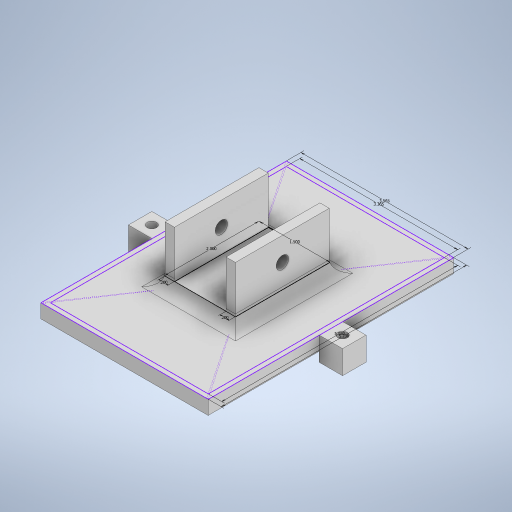
# Autodesk Inventor part: HotplateRetainer for 8020
Saved by Autodesk Inventor 2024.1 (Build 281209000, 209)
## iProperties
Created: 2022-02-14
Part Number: HotplateRetainer for 8020
Material: Generic
Document SubType Name: Modeling
Designer: Beaucage
Density: 1 g/cm^3
Appearance: Default
Author: Beaucage
Autodesk Inventor part; units mm, degrees
ref_plane "YZ Plane" through (0, 0, 0) normal (1, 0, 0) x (0, 1, 0)
ref_plane "XZ Plane" through (0, 0, 0) normal (0, 1, 0) x (-1, 0, 0)
ref_plane "XY Plane" through (0, 0, 0) normal (0, 0, 1) x (1, 0, 0)
sketch "Sketch1" plane through (0, 0, 0) normal (0, 1, 0) x (-1, 0, 0)
  line L0 (0, 0) -> (38.1, 0)
  line L1 (38.1, 0) -> (38.1, -50.8)
  line L2 (38.1, -50.8) -> (0, -50.8)
  line L3 (0, -50.8) -> (0, 0)
  line L4 (38.1, -50.8) -> (33.02, -50.8)
  line L5 (33.02, -50.8) -> (33.02, 0)
  line L6 (33.02, 0) -> (38.1, 0)
  line L7 (38.1, 0) -> (38.1, -50.8)
  line L8 (0, -50.8) -> (5.08, -50.8)
  line L9 (5.08, -50.8) -> (5.08, 0)
  line L10 (5.08, 0) -> (0, 0)
  line L11 (0, 0) -> (0, -50.8)
  dimension "d0" = 38.1
  dimension "d1" = 50.8
  dimension "d2" = 5.08
  dimension "d3" = 5.08
  constraints: 24 end point, 6 parallel, 3 horizontal, 3 perpendicular, 2 point on line
  measures "d0" distance of L1.end L2.end
  measures "d1" distance of L0.end L1.end
  measures "d2" distance of L5.end L6.end
  measures "d3" distance of L10.end L9.end
extrude "Extrusion1" add sketch "Sketch1" along normal blind 25.4 contours L0 L9 L2 L3 | L0 L1 L2 L5
extrude "Extrusion2" add sketch "Sketch1" against normal blind 5.08
sketch "Sketch2" plane through (0, 25.4, 0) normal (1, 0, 0) x (0, 0, -1)
  line L0 (50.8, 0) -> (0, 0) projected
  line L1 (25.4, 0) -> (25.4, -12.7)
  point P0 (0, -25.4)
  dimension "d8" = 12.7
  constraints: 2 end point, 1 midpoint, 1 vertical
  measures "d8" distance of L1.start L1.end
hole "Hole1" at (0, 12.7, -25.4) direction (-1, 0, 0) diameter 6.7564 end through all start extended yes clearance for "Socket Head Cap Screw" size "1/4" standard "Ansi Unified Screw Threads"
sketch "Sketch3" plane through (0, -5.08, 0) normal (0, -1, 0) x (1, 0, 0)
  line L0 (0, 0) -> (-38.1, 0) projected
  line L1 (-38.1, 0) -> (-38.1, -50.8) projected
  line L2 (-38.1, -50.8) -> (0, -50.8) projected
  line L3 (0, -50.8) -> (0, 0) projected
  line L4 (-61.7906, 38.4797) -> (23.6906, 38.4797)
  line L5 (23.6906, 38.4797) -> (23.6906, -89.2797)
  line L6 (23.6906, -89.2797) -> (-61.7906, -89.2797)
  line L7 (-61.7906, -89.2797) -> (-61.7906, 38.4797)
  line L8 (-61.7906, 38.4797) -> (23.6906, -89.2797) construction
  line L9 (23.6906, 38.4797) -> (-61.7906, -89.2797) construction
  line L10 (-63.4909, 41.021) -> (25.3909, 41.021)
  line L11 (25.3909, -91.821) -> (-63.4909, -91.821)
  line L12 (-63.4909, 41.021) -> (25.3909, -91.821) construction
  line L13 (25.3909, 41.021) -> (-63.4909, -91.821) construction
  line L14 (-64.3255, 41.021) -> (26.2255, 41.021)
  line L15 (26.2255, 41.021) -> (26.2255, -91.821)
  line L16 (26.2255, -91.821) -> (-64.3255, -91.821)
  line L17 (-64.3255, -91.821) -> (-64.3255, 41.021)
  line L18 (-64.3255, 41.021) -> (26.2255, -91.821) construction
  line L19 (26.2255, 41.021) -> (-64.3255, -91.821) construction
  point P0 (-19.05, -25.4)
  point P1 (25.3909, 41.021)
  dimension "d16" = 85.4812
  dimension "d17" = 127.7595
  dimension "d18" = 132.842
  dimension "d19" = 90.551
  constraints: 32 end point, 6 midpoint, 5 parallel, 3 horizontal, 2 perpendicular
  measures "d16" distance of L5.end L6.end
  measures "d17" distance of L4.end L5.end
  measures "d18" distance of L10.end L11.start
  measures "d19" distance of L15.end L16.end
extrude "Extrusion3" add sketch "Sketch3" along normal blind 2.54 contours L3 L2 L1 L0 | L4 L5 L6 L7
extrude "Extrusion4" add sketch "Sketch3" along normal blind 7.62 contours L10 L14 L15 L16 L11 L17
fillet "Fillet1" radius 6.35 4 edges at (-38.1, -5.08, -25.4) (-19.05, -5.08, -50.8) (0, -5.08, -25.4) (-19.05, -5.08, 0)
sketch "Sketch4" plane through (0, -5.08, 0) normal (0, 1, 0) x (1, 0, 0)
  line L0 (-51.6255, 19.05) -> (-77.0255, 19.05)
  line L1 (-77.0255, 19.05) -> (-77.0255, 31.75)
  line L2 (-77.0255, 31.75) -> (-51.6255, 31.75)
  line L3 (-51.6255, 31.75) -> (-51.6255, 19.05)
  line L4 (-64.3255, -41.021) -> (-64.3255, 91.821) projected
  line L5 (-51.6255, 19.05) -> (-77.0255, 31.75) construction
  line L6 (-77.0255, 19.05) -> (-51.6255, 31.75) construction
  line L7 (13.5255, 19.05) -> (38.9255, 19.05)
  line L8 (38.9255, 19.05) -> (38.9255, 31.75)
  line L9 (38.9255, 31.75) -> (13.5255, 31.75)
  line L10 (13.5255, 31.75) -> (13.5255, 19.05)
  line L11 (26.2255, 91.821) -> (26.2255, -41.021) projected
  line L12 (13.5255, 19.05) -> (38.9255, 31.75) construction
  line L13 (38.9255, 19.05) -> (13.5255, 31.75) construction
  point P0 (0, 0)
  point P1 (-64.3255, 25.4)
  point P2 (26.2255, 25.4)
  point P3 (26.2255, 31.75)
  point P4 (26.2255, 19.05)
  point P5 (-64.3255, 19.05)
  point P6 (-64.3255, 31.75)
  dimension "d25" = 25.4
  dimension "d26" = 12.7
  dimension "d27" = 25.4
  dimension "d28" = 12.7
  constraints: 24 end point, 6 midpoint, 4 parallel, 2 horizontal, 2 perpendicular
  measures "d25" distance of L1.end L2.end
  measures "d26" distance of L0.end L1.end
  measures "d27" distance of L9.end L8.end
  measures "d28" distance of L8.end L7.end
extrude "Extrusion5" add sketch "Sketch4" against normal blind 12.7 contours L0 L1 L2 L4 | L11 L9 L8 L7
sketch "Sketch5" plane through (0, -17.78, 0) normal (0, -1, 0) x (1, 0, 0)
  line L0 (26.2255, -31.75) -> (38.9255, -31.75) projected
  line L1 (38.9255, -31.75) -> (38.9255, -19.05) projected
  line L2 (38.9255, -19.05) -> (26.2255, -19.05) projected
  line L3 (26.2255, -19.05) -> (26.2255, -31.75) projected
  line L4 (-64.3255, -19.05) -> (-77.0255, -19.05) projected
  line L5 (-77.0255, -19.05) -> (-77.0255, -31.75) projected
  line L6 (-77.0255, -31.75) -> (-64.3255, -31.75) projected
  line L7 (-64.3255, -31.75) -> (-64.3255, -19.05) projected
  point P0 (0, 0)
  point P1 (32.5755, -25.4)
  point P2 (-70.6755, -25.4)
hole "Hole2" at (32.5755, -17.78, -25.4) at (-70.6755, -17.78, -25.4) direction (0, 1, 0) diameter 5.1594 end through all
body "Solid1"
